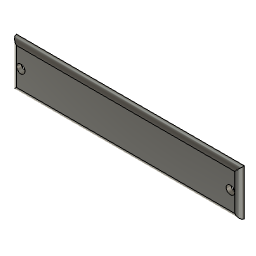
Obere heckplatte (Autodesk Fusion 360 design; units mm, degrees)
Autodesk Fusion 360 part; units mm, degrees
sketch "Skizze1" plane through (0, 0, 0) normal (0, 1, 0) x (1, 0, 0)
  line L0 (0, 0) -> (94, 0)
  line L1 (0, 0) -> (0, -19)
  line L2 (0, -19) -> (94, -19)
  line L3 (94, -19) -> (94, 0)
  dimension "d1" = 94
  dimension "d2" = 19
  constraint coincident L0.start L1.start
  constraint horizontal L0
  constraint perpendicular L0 L1
  constraint perpendicular L1 L2
  constraint perpendicular L0 L3
  measures "d1" distance of L0.start L0.end
  measures "d2" distance of L0.start L1.end
extrude "Extrusion1" add sketch "Skizze1" along normal blind 2
sketch "Skizze2" plane through (0, 0, 0) normal (0, -1, 0) x (1, 0, 0)
  line L0 (0, 19) -> (0, 0)
  line L1 (0, 0) -> (94, 0)
  line L2 (94, 0) -> (94, 19)
  line L3 (94, 19) -> (0, 19)
  circle A0 centre (3.75, 9.5) radius 1.75
  circle A1 centre (90.25, 9.5) radius 1.75
  dimension "d8" = 3.5
  dimension "d9" = 3.5
  measures "d8" diameter of A0
  measures "d9" diameter of A1
extrude "Extrusion2" cut sketch "Skizze2" against normal blind 2 contours A0 | A1
fillet "Abrundung1" radius 2 4 edges at (47, 0, 19) (94, 0, 9.5) (47, 0, 0) (0, 0, 9.5)
